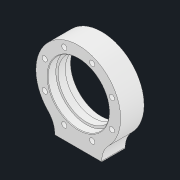
# Autodesk Inventor part: scara-base15
Saved by Autodesk Inventor 2022 (Build 260153000, 153)
## iProperties
Created: 2021-10-12
Part Number: scara-base15
Material: ABS プラスチック
Document SubType Name: Modeling
Designer: Yuta Kage
Density: 1.06 g/cm^3
Appearance: 滑らか - 白
Description: 印刷
Mass: 46.1133 g
Surface Area: 150.511 cm^2
Volume: 43.5031 cm^3
Author: Yuta Kage
Autodesk Inventor part; units mm, degrees
ref_plane "YZ Plane" through (0, 0, 0) normal (1, 0, 0) x (0, 1, 0)
ref_plane "XZ Plane" through (0, 0, 0) normal (0, 1, 0) x (-1, 0, 0)
ref_plane "XY Plane" through (0, 0, 0) normal (0, 0, 1) x (1, 0, 0)
sketch "スケッチ1" plane through (0, 0, 0) normal (1, 0, 0) x (0, 1, 0)
  line L0 (26.1, 0) -> (36.1, 0)
  line L1 (36.1, 0) -> (36.1, 20)
  line L2 (36.1, 20) -> (26.1, 20)
  line L3 (26.1, 20) -> (26.1, 13.05)
  line L4 (26.1, 13.05) -> (24.1, 13.05)
  line L5 (0, -4) -> (0, 24) projected
  line L6 (24.1, 13.05) -> (24.1, 6.95)
  line L7 (24.1, 6.95) -> (26.1, 6.95)
  line L8 (26.1, 6.95) -> (26.1, 0)
  point P0 (0, 0)
  dimension "d0" = 26.1
  dimension "d2" = 6.95
  dimension "d3" = 20
  dimension "d4" = 10
  dimension "d28" = 2
  dimension "d29" = 6.95
  constraints: 16 end point, 6 perpendicular, 1 horizontal, 1 horizontal alignment, 1 vertical, 1 vertical alignment
  measures "d0" distance from line of point (0, 0) L3
  measures "d2" distance of L2.end L3.end
  measures "d3" distance of L0.end L1.end
  measures "d4" distance of L1.end L2.end
  measures "d28" distance of L3.end L4.end
  measures "d29" distance of L7.end L0.start
revolve "回転1" add sketch "スケッチ1" angle 360 about axis through (0, 0, -10) along (0, 0, 1)
sketch "スケッチ2" plane through (0, 0, 0) normal (0, 0, -1) x (-1, 0, 0)
  circle A0 centre (0, 0) radius 31
  point P0 (-11.8632, 28.6403)
  point P1 (-28.6403, 11.8632)
  point P2 (-28.6403, -11.8632)
  point P3 (-11.8632, -28.6403)
  point P4 (11.8632, -28.6403)
  point P5 (28.6403, -11.8632)
  point P6 (28.6403, 11.8632)
  point P7 (11.8632, 28.6403)
  dimension "d6" = 62
  dimension "d9" = 360
  dimension "d25" = 0
  constraints: 1 coincident, 12 other
  measures "d25" vertical distance of point (11.863, 28.64) point (-11.863, 28.64)
hole "穴1" at (11.8632, 28.6403, 0) at (28.6403, 11.8632, 0) at (28.6403, -11.8632, 0) at (11.8632, -28.6403, 0) at (-11.8632, -28.6403, 0) at (-28.6403, -11.8632, 0) at (-28.6403, 11.8632, 0) at (-11.8632, 28.6403, 0) direction (0, 0, 1) diameter 4.5 end through all clearance for "Flat Head Machine Screw" size "M4" standard "Ansi Metric M Profile"
chamfer "面取り1" distance 0.5 angle 45 2 edges at (0, -26.1, 20) (0, -26.1, 0)
sketch "スケッチ3" plane through (0, 0, 0) normal (0, 0, -1) x (-1, 0, 0)
  line L0 (-20, -30.0535) -> (20, -30.0535)
  line L1 (20, -30.0535) -> (20, -40)
  line L2 (20, -40) -> (-20, -40)
  line L3 (-20, -40) -> (-20, -30.0535)
  line L4 (-20, -30.0535) -> (20, -40) construction
  line L5 (20, -30.0535) -> (-20, -40) construction
  circle A0 centre (0, 0) radius 36.1 projected
  point P0 (0, -35.0267)
  point P1 (0, -35.0267)
  point P2 (20, -30.0535)
  dimension "d21" = 40
  dimension "d22" = 40
  constraints: 12 end point, 3 midpoint, 2 parallel, 1 horizontal, 1 perpendicular, 1 vertical alignment, 2 other
  measures "d21" distance from line of point (0, 0) L2
  measures "d22" distance of L1.end L2.end
extrude "押し出し1" add sketch "スケッチ3" against normal up to surface (20 mm away) contours A0 L1 L2 L3
fillet "フィレット2" radius 20 2 edges at (20, -30.0535, 10) (-20, -30.0535, 10)
equation "\"d29\" = d2"
